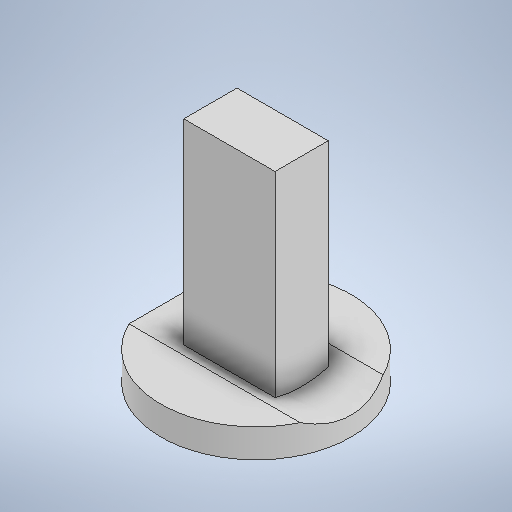
# Autodesk Inventor part: Pin
Saved by Autodesk Inventor 2026.2 (Build 302298010, 298A)
## iProperties
Created: 2026-05-05
Part Number: Pin
Material: Generic
Document SubType Name: Modeling
Designer: piete
Density: 1 g/cm^3
Appearance: Default
Author: piete
Autodesk Inventor part; units mm, degrees
ref_plane "YZ Plane" through (0, 0, 0) normal (1, 0, 0) x (0, 1, 0)
ref_plane "XZ Plane" through (0, 0, 0) normal (0, 1, 0) x (-1, 0, 0)
ref_plane "XY Plane" through (0, 0, 0) normal (0, 0, 1) x (1, 0, 0)
sketch "Sketch1" plane through (0, 0, 0) normal (0, 1, 0) x (-1, 0, 0)
  line L0 (4.9, 2.9) -> (-4.9, 2.9)
  line L1 (-4.9, 2.9) -> (-4.9, -2.9)
  line L2 (-4.9, -2.9) -> (4.9, -2.9)
  line L3 (4.9, -2.9) -> (4.9, 2.9)
  point P0 (0, 0)
  dimension "d0" = 9.8
  dimension "d1" = 5.8
  dimension "d2" = 2.9
  dimension "d3" = 4.9
  constraints: 8 end point, 2 parallel, 1 horizontal, 1 perpendicular
  measures "d0" distance of L2.end L1.end
  measures "d1" distance of L1.end L0.end
  measures "d2" distance from line of point (0, 0) L2
  measures "d3" distance from line of point (0, 0) L1
extrude "Extrusion1" add sketch "Sketch1" along normal blind 20
sketch "Sketch2" plane through (0, 0, 0) normal (0, -1, 0) x (1, 0, 0)
  circle A0 centre (0, 0) radius 10
  dimension "d6" = 20
  constraints: 1 centre point, 1 coincident
  measures "d6" diameter of A0
extrude "Extrusion2" add sketch "Sketch2" along normal blind 3
sketch "Sketch3" plane through (0, 20, 0) normal (0, 1, 0) x (1, 0, 0)
  line L0 (-4.9, 2.9) -> (-4.9, -2.9) projected
  line L1 (-4.9, -2.9) -> (4.9, -2.9) projected
  line L2 (-4.9, 2.9) -> (4.9, 2.9)
  line L3 (4.9, 2.9) -> (4.9, -2.9)
  line L4 (4.9, -2.9) -> (-4.9, -2.9)
  line L5 (-4.9, -2.9) -> (-4.9, 2.9)
  point P0 (0, 0)
  constraints: 8 end point, 2 parallel, 1 horizontal, 1 perpendicular
extrude "Extrusion3" cut sketch "Sketch3" against normal up to surface (20 mm away)
sketch "Sketch4" plane through (0, 0, 0) normal (1, 0, 0) x (0, 1, 0)
  circle A0 centre (9, 0) radius 10
  line L0 (-3, 10) -> (-3, -10) projected
  point P0 (0, 0)
  point P1 (-3, 0)
  dimension "d11" = 20
  dimension "d12" = 12
  dimension "d13" = 0
  constraints: 1 centre point, 1 midpoint
  measures "d11" diameter of A0
  measures "d12" distance from line of L0 A0.centre
  measures "d13" vertical distance of point (-3, 0) A0.centre
extrude "Extrusion4" cut sketch "Sketch4" along normal through all both and the other way through all
sketch "Sketch5" plane through (0, -3, 0) normal (0, -1, 0) x (1, 0, 0)
  line L0 (-4.8, 2.8) -> (4.8, 2.8)
  line L1 (4.8, 2.8) -> (4.8, -2.8)
  line L2 (4.8, -2.8) -> (-4.8, -2.8)
  line L3 (-4.8, -2.8) -> (-4.8, 2.8)
  point P0 (0, 0)
  dimension "d16" = 9.6
  dimension "d17" = 5.6
  dimension "d18" = 2.8
  dimension "d19" = 4.8
  constraints: 8 end point, 2 parallel, 1 horizontal, 1 perpendicular
  measures "d16" distance of L1.end L2.end
  measures "d17" distance of L0.end L1.end
  measures "d18" distance from line of point (0, 0) L0
  measures "d19" distance from line of L1 point (0, 0)
extrude "Extrusion5" add sketch "Sketch5" against normal blind 23
equation "\"d2\" = 0.5 * d1"
equation "\"d3\" = 0.5 * d0"
equation "\"d18\" = 0.5 * d17"
equation "\"d19\" = 0.5 * d16"
body "Solid1"
